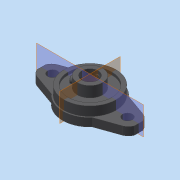
# Autodesk Inventor part: UFL08 -Housing
Saved by Autodesk Inventor 2016 SP1 (Build 200210100, 210)
## iProperties
Category: PARTsolutions
Company: NIPPON_PB
Created: 2015-11-15
Part Number: UFL08 -Housing
Catalog Web Link: www.cadenas.de
Description: CS RFU with Setscrew Housing-Housing
Vendor: NIPPON_PB
Document SubType Name: Modeling
Designer: psAdmin
Manufacturer: NIPPON_PB
Mass: 4.71693 g
Surface Area: 32.0343 cm^2
Volume: 4.71693 cm^3
Density: 1 g/cm^3
Material: Generic
Appearance: PSOLRGB-192-192-192
PSOL_IDENT_0: {$CADENAS_DATA\23d-libs\nippon_pb\clean_series\rhombic_flange_unit\parts\cs_rfu_with_setscrew_housin
PSOL_IDENT_1: g.prj},198 {VTYP=3D},{NB=UFL08 -Housing},{LINA=UFL08 -Housing},{NN=CS RFU with Setscrew Housing},{DA
PSOL_IDENT_2: TE=08.05.2013 00:57:51},{GEOMDATE=27.08.2007 08:16:00},{VERSION=},{LINEID=10},{LINESUBID=-1},{WBVAR=
PSOL_IDENT_3: C,TOCE}  {NB=UFL08 -Housing},{LINA=UFL08 -Housing},{KT=DUMMY},{D=8.000},{C=},{TOCE= },{G=3.000},{S2=
PSOL_IDENT_4: 3.000},{S5=1.500},{H=48.000},{L=27.000},{A=8.500},{J=37.000},{N=4.800},{A1=4.000},{A2=4.000},{A0=12.
PSOL_IDENT_5: 500},{B=12.000},{S=3.500},{UN=UFL08},{AS=0.000},{D6=12.400},{R=5.500},{R1=0.000},{J1=0.000},{D7=14.0
PSOL_IDENT_6: 00},{J2=0.000},{J3=0.430},{C1= '','without cover' },{C2= ' ','None' }
NN: CS RFU with Setscrew Housing
NT: Housing
NB: UFL08 -Housing
NBSYN: $UN.$C.$TOCE.-Housing
LINA: UFL08 -Housing
D: 8.000
C: without cover
G: 3.000
S2: 3.000
S5: 1.500
H: 48.000
L: 27.000
A: 8.500
J: 37.000
N: 4.800
A1: 4.000
A2: 4.000
A0: 12.500
B: 12.000
S: 3.500
UN: UFL08
AS: 0.000
D6: 12.400
R: 5.500
R1: 0.000
J1: 0.000
D7: 14.000
J2: 0.000
J3: 0.430
SUPPLIER: NIPPON_PB
ARTICLENO: UFL08 -Housing
BOMINFO: UFL08 -Housing
CREATOR: CADENAS GmbH
Title: UFL08 -Housing
Author: Cadenas PARTsolutions
Comments: Housing
Autodesk Inventor part; units mm, degrees
ref_plane "YZ Plane" through (0, 0, 0) normal (1, 0, 0) x (0, 1, 0)
ref_plane "XZ Plane" through (0, 0, 0) normal (0, 1, 0) x (-1, 0, 0)
sketch "Sketch_1" plane through (0, 0, 0) normal (0, 0, 1) x (1, 0, 0)
  line L0 (-24, 2.1319) -> (-24, -2.1319)
  arc A0 (-24, -2.1319) -> (-21.25, -4.9867) centre (-18.93, 0) ccw
  line L1 (-21.25, -4.9867) -> (-10.125, -8.9294)
  arc A1 (-10.125, -8.9294) -> (10.125, -8.9294) centre (0, 0) ccw
  line L2 (10.125, -8.9294) -> (21.25, -4.9867)
  arc A2 (21.25, -4.9867) -> (24, -2.1319) centre (18.93, 0) ccw
  line L3 (24, -2.1319) -> (24, 2.1319)
  arc A3 (24, 2.1319) -> (21.25, 4.9867) centre (18.93, 0) ccw
  line L4 (21.25, 4.9867) -> (10.125, 8.9294)
  arc A4 (10.125, 8.9294) -> (-10.125, 8.9294) centre (0, 0) ccw
  line L5 (-10.125, 8.9294) -> (-21.25, 4.9867)
  arc A5 (-21.25, 4.9867) -> (-24, 2.1319) centre (-18.93, 0) ccw
  circle A6 centre (18.5, 0) radius 2.4
  circle A7 centre (0, 0) radius 6.2
  circle A8 centre (-18.5, 0) radius 2.4
  constraints: 12 end point, 12 point on circle, 9 centre point
extrude "Extrusion1" add sketch "Sketch_1" along normal blind 4
sketch "Sketch_2" plane through (0, 0, 0) normal (1, 0, 0) x (0, 1, 0)
  line L0 (0, 0) -> (0, 8.5)
  line L1 (12.825, 8.5) -> (10.8, 8.5)
  line L2 (10.8, 8.5) -> (10.8, 7.225)
  line L3 (10.8, 7.225) -> (6.2, 7.225)
  line L4 (6.2, 7.225) -> (6.2, 0)
  line L5 (6.2, 0) -> (12.825, 0)
  line L6 (12.825, 0) -> (12.825, 8.5)
  constraints: 14 end point
revolve "Revolution1" add sketch "Sketch_2" angle 360 about axis through (0, 0, 0) along (0, 0, -1)
sketch "Sketch_5" plane through (0, 0, 0) normal (0, 0, 1) x (1, 0, 0)
  circle A0 centre (0, 0) radius 12.15
  constraints: 1 centre point
extrude "Extrusion2" cut sketch "Sketch_5" along normal blind 1
sketch "Sketch_6" plane through (0, 0, 0) normal (1, 0, 0) x (0, 1, 0)
  line L0 (0, -27) -> (0, 27)
  line L1 (6.2, 12.5) -> (4, 12.5)
  line L2 (4, 12.5) -> (4, 0.5)
  line L3 (4, 0.5) -> (6.2, 0.5)
  line L4 (6.2, 0.5) -> (6.2, 12.5)
  constraints: 10 end point
revolve "Revolution2" add sketch "Sketch_6" angle 360 about axis through (0, 0, -27) along (0, 0, -1)
sketch "Sketch_7" plane through (0, 0, 9.5) normal (0, 0, 1) x (1, 0, 0)
  line L0 (0, 0) -> (0, 6.2)
  line L1 (0, 6.2) -> (1.5, 6.2)
  line L2 (1.5, 6.2) -> (1.5, 0)
  line L3 (1.5, 0) -> (0, 0)
  line L4 (0, 0) -> (0, 6.2)
  constraints: 10 end point
revolve "Revolution3" cut sketch "Sketch_7" angle 360 about axis through (0, 0, 9.5) along (0, -1, 0)
sketch "Sketch_8" plane through (0, 0, 9.5) normal (0, 0, 1) x (1, 0, 0)
  line L0 (0, 0) -> (-5.3694, -3.1)
  line L1 (-5.3694, -3.1) -> (-6.1194, -1.801)
  line L2 (-6.1194, -1.801) -> (-0.75, 1.299)
  line L3 (-0.75, 1.299) -> (0, 0)
  line L4 (0, 0) -> (-5.3694, -3.1)
  constraints: 10 end point
revolve "Revolution4" cut sketch "Sketch_8" angle 360 about axis through (0, 0, 9.5) along (0.8660254, 0.5, 0)
sketch "Sketch_9" plane through (0, 0, 9.5) normal (0, 0, 1) x (1, 0, 0)
  line L0 (0, 4) -> (0, 4.8775)
  line L1 (0, 4.8775) -> (0.9225, 5.8)
  line L2 (0.9225, 5.8) -> (0.9225, 7)
  line L3 (0.9225, 7) -> (1.436, 7)
  arc A0 (1.5, 6.936) -> (1.436, 7) centre (1.436, 6.936) ccw
  line L4 (1.5, 6.936) -> (1.5, 4.5)
  line L5 (1.5, 4.5) -> (1, 4)
  line L6 (1, 4) -> (0, 4)
  line L7 (0, 4) -> (0, 4.8775)
  constraints: 16 end point, 2 point on circle, 1 centre point
revolve "Revolution5" add sketch "Sketch_9" angle 360 about axis through (0, 4, 9.5) along (0, -1, 0)
sketch "Sketch_10" plane through (0, 0, 9.5) normal (0, 0, 1) x (1, 0, 0)
  line L0 (-3.4641, -2) -> (-4.224, -2.4388)
  line L1 (-4.224, -2.4388) -> (-5.4842, -2.1011)
  line L2 (-5.4842, -2.1011) -> (-6.5234, -2.7011)
  line L3 (-6.5234, -2.7011) -> (-6.7802, -2.2564)
  arc A0 (-6.7568, -2.169) -> (-6.7802, -2.2564) centre (-6.7248, -2.2244) ccw
  line L4 (-6.7568, -2.169) -> (-4.6471, -0.951)
  line L5 (-4.6471, -0.951) -> (-3.9641, -1.134)
  line L6 (-3.9641, -1.134) -> (-3.4641, -2)
  line L7 (-3.4641, -2) -> (-4.224, -2.4388)
  constraints: 16 end point, 2 point on circle, 1 centre point
revolve "Revolution6" add sketch "Sketch_10" angle 360 about axis through (-3.4641, -2, 9.5) along (0.8660254, 0.5, 0)
sketch "Sketch_11" plane through (0, 7, 0) normal (0, 1, 0) x (1, 0, 0)
  line L0 (-0.975, -8.6195) -> (-0.975, -10.3805)
  line L1 (-0.975, -10.3805) -> (-0.8113, -10.475)
  line L2 (-0.8113, -10.475) -> (0.8113, -10.475)
  line L3 (0.8113, -10.475) -> (0.975, -10.3805)
  line L4 (0.975, -10.3805) -> (0.975, -8.6195)
  line L5 (0.975, -8.6195) -> (0.8113, -8.525)
  line L6 (0.8113, -8.525) -> (-0.8113, -8.525)
  line L7 (-0.8113, -8.525) -> (-0.975, -8.6195)
  line L8 (-0.75, -9.933) -> (0, -10.366)
  line L9 (0, -10.366) -> (0.75, -9.933)
  line L10 (0.75, -9.933) -> (0.75, -9.067)
  line L11 (0.75, -9.067) -> (0, -8.634)
  line L12 (0, -8.634) -> (-0.75, -9.067)
  line L13 (-0.75, -9.067) -> (-0.75, -9.933)
  constraints: 28 end point
extrude "Extrusion3" add sketch "Sketch_11" against normal blind 1.5
sketch "Sketch_12" plane through (-6.0622, -3.5, 0) normal (0.8660254, 0.5, 0) x (0.5, -0.8660254, 0)
  line L0 (-0.975, -8.6195) -> (-0.975, -10.3805)
  line L1 (-0.975, -10.3805) -> (-0.8113, -10.475)
  line L2 (-0.8113, -10.475) -> (0.8113, -10.475)
  line L3 (0.8113, -10.475) -> (0.975, -10.3805)
  line L4 (0.975, -10.3805) -> (0.975, -8.6195)
  line L5 (0.975, -8.6195) -> (0.8113, -8.525)
  line L6 (0.8113, -8.525) -> (-0.8113, -8.525)
  line L7 (-0.8113, -8.525) -> (-0.975, -8.6195)
  line L8 (-0.75, -9.933) -> (0, -10.366)
  line L9 (0, -10.366) -> (0.75, -9.933)
  line L10 (0.75, -9.933) -> (0.75, -9.067)
  line L11 (0.75, -9.067) -> (0, -8.634)
  line L12 (0, -8.634) -> (-0.75, -9.067)
  line L13 (-0.75, -9.067) -> (-0.75, -9.933)
  constraints: 28 end point
extrude "Extrusion4" add sketch "Sketch_12" along normal blind 1.5
ref_plane "housing_XY" through (-18.5, 0, 0) normal (0, 0, 1) x (1, 0, 0)
ref_plane "housing_YZ" through (-18.5, 0, 0) normal (1, 0, 0) x (0, 1, 0)
ref_plane "housing_ZX" through (-18.5, 0, 0) normal (0, 1, 0) x (0, 0, 1)
ref_plane "Work Plane4" through (0, 13.5, 4) normal (1, 0, 0) x (0, 1, 0)
ref_plane "Work Plane5" through (24, 0, 4) normal (0, 1, 0) x (0, 0, 1)
body "Solid1"
